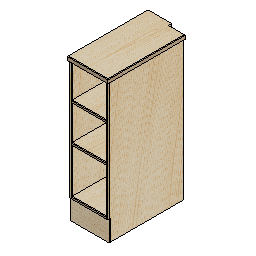
model (Autodesk Fusion 360 design; units mm, degrees)
Autodesk Fusion 360 part; units mm, degrees
note: some values were not read from the file. Chosen so that the rebuilt part matches the saved one: which bodies a step acts on.
sketch "cabinet" plane through (0, 0, 0) normal (1, 0, 0) x (0, 1, 0) in component "bounds"
  line L0 (0, 0) -> (0, 109)
  line L1 (0, 109) -> (-72, 109)
  line L2 (-72, 109) -> (-72, 884)
  line L3 (-72, 884) -> (413, 884)
  line L4 (413, 884) -> (413, 0)
  line L5 (413, 0) -> (0, 0)
  line L6 (-72, 884) -> (-102, 884)
  line L7 (-102, 884) -> (-102, 914)
  line L8 (-102, 914) -> (413, 914)
  line L9 (413, 914) -> (413, 884)
  dimension "d1" = 30
  dimension "d2" = 30
  dimension "d3" = 109
  dimension "d4" = 72
  dimension "d5" = 485
  dimension "d6" = 884
  constraint coincident L0.start L5.end
  constraint vertical L0
  constraint horizontal L1
  constraint vertical L2
  constraint horizontal L5
  constraint vertical L4
  constraint horizontal L3
  constraint vertical L9
  constraint horizontal L6
  constraint vertical L7
  constraint horizontal L8
  measures "d1" distance of L2.end L6.end
  measures "d2" distance of L6.end L7.end
  measures "d3" distance of L0.start L0.end
  measures "d4" distance of L0.end L1.end
  measures "d5" distance of L2 L4
  measures "d6" distance of L3.end L4.end
extrude "Extrude1" add sketch "cabinet" against normal blind 30 makes body 1 in component "bounds"
extrude "Extrude2" add sketch "cabinet" along normal blind 30 contours L3 L6 L7 L8 L9 bodies 1 in component "bounds"
sketch "wall" plane through (0, 413, 0) normal (0, 1, 0) x (-1, 0, 0) in component "bounds"
  line L0 (0, 884) -> (0, 0)
  line L1 (0, 0) -> (30, 0)
  line L2 (30, 0) -> (30, 914)
  line L3 (30, 914) -> (-30, 914)
  line L4 (-30, 914) -> (-30, 884)
  line L5 (-30, 884) -> (0, 884)
  line L6 (30, 914) -> (-205, 914)
  line L7 (-205, 914) -> (-205, 0)
  line L8 (-205, 0) -> (30, 0)
  line L9 (30, 0) -> (30, 914)
  line L10 (-127, 914) -> (-127, 95)
  line L11 (-127, 95) -> (0, 95)
  dimension "d11" = 78
  dimension "d13" = 95
  dimension "d14" = 205
  constraint horizontal L6
  constraint vertical L7
  constraint horizontal L8
  constraint vertical L9
  constraint coincident L2.end L3.start
  constraint coincident L0.end L8
  constraint coincident L6 L10.start
  constraint coincident L0 L11.end
  constraint vertical L10
  constraint horizontal L11
  measures "d11" distance of L7 L10
  measures "d13" distance of L8 L11
  measures "d14" distance of L0 L7
extrude "Extrude3" add sketch "wall" along normal blind 30 separate body makes body 2 in component "bounds"
extrude "Extrude4" add sketch "wall" against normal blind 18 contours L0 L6 L7 L8 L10 L11 bodies 2 in component "bounds"
sketch "bathtub" plane through (205, 0, 0) normal (1, 0, 0) x (0, 1, 0) in component "bounds"
  line L0 (395, 0) -> (443, 0)
  line L1 (443, 0) -> (443, 914)
  line L2 (443, 914) -> (395, 914)
  line L3 (395, 914) -> (395, 0)
  line L4 (443, 0) -> (-357, 0)
  line L5 (-357, 0) -> (-357, 520)
  line L6 (-357, 520) -> (443, 520)
  line L7 (443, 520) -> (443, 0)
  dimension "d19" = 520
  dimension "d20" = 800
  constraint horizontal L4
  constraint vertical L5
  constraint horizontal L6
  constraint vertical L7
  constraint coincident L0.end L1.start
  measures "d19" distance of L4.end L5.end
  measures "d20" distance of L0.end L4.end
extrude "Extrude5" add sketch "bathtub" along normal blind 30 separate body contours L0 L1 L3 L4 L6 L7 | L3 L4 L5 L6 makes body 3 in component "bounds"
extrude "Extrude6" add sketch "bathtub" along normal blind 30 contours L1 L2 L3 L6 bodies 2 in component "bounds"
sketch "face" plane through (0, 0, 0) normal (0, 1, 0) x (1, 0, 0) in component "unit"
  line L0 (0, 0) -> (205, 0)
  line L1 (205, 0) -> (205, -750)
  line L2 (205, -750) -> (0, -750)
  line L3 (0, -750) -> (0, 0)
  line L4 (9, -750) -> (9, 0)
  line L5 (196, -750) -> (196, 0)
  line L6 (9, -375) -> (0, -375) construction
  line L7 (205, -375) -> (196, -375) construction
  line L8 (0, -750) -> (0, -768)
  line L9 (0, -768) -> (217, -768)
  line L10 (205, -750) -> (217, -750)
  line L11 (217, -750) -> (217, -768)
  line L12 (9, -118) -> (196, -118)
  line L13 (196, -109) -> (9, -109)
  line L14 (0, -109) -> (-30, -109)
  line L15 (196, -109) -> (205, -109)
  line L16 (9, -109) -> (0, -109)
  line L17 (9, -563) -> (196, -563)
  line L18 (196, -554) -> (9, -554)
  line L19 (9, -367) -> (196, -367)
  line L20 (196, -358) -> (9, -358)
  dimension "d25" = 205
  dimension "d26" = 9
  dimension "d27" = 750
  dimension "d32" = 18
  dimension "d33" = 12
  dimension "d34" = 9
  dimension "d35" = 9
  dimension "d36" = 187
  dimension "d37" = 9
  dimension "d38" = 187
  dimension "d39" = 240
  constraint horizontal L0
  constraint vertical L1
  constraint horizontal L2
  constraint vertical L3
  constraint coincident L0.start L3.end
  constraint coincident L2 L4.start
  constraint coincident L2 L5.start
  constraint coincident L0 L5.end
  constraint vertical L4
  constraint vertical L5
  constraint coincident L0 L4.end
  constraint midpoint L4 L6.start
  constraint midpoint L3 L6.end
  constraint midpoint L1 L7.start
  constraint midpoint L5 L7.end
  constraint equal L6 L7
  constraint vertical L8
  constraint horizontal L9
  constraint horizontal L10
  constraint vertical L11
  constraint coincident L4 L12.start
  constraint coincident L5 L12.end
  constraint coincident L5 L13.start
  constraint coincident L4 L13.end
  constraint horizontal L13
  constraint horizontal L12
  constraint coincident L1 L15.end
  constraint perpendicular L1 L15
  constraint coincident L3 L14.start
  constraint perpendicular L3 L16
  constraint coincident L4 L17.start
  constraint coincident L5 L17.end
  constraint coincident L5 L18.start
  constraint coincident L4 L18.end
  constraint horizontal L18
  constraint horizontal L17
  constraint coincident L4 L19.start
  constraint coincident L5 L19.end
  constraint coincident L5 L20.start
  constraint coincident L4 L20.end
  constraint horizontal L20
  constraint horizontal L19
  constraint collinear L13 L14
  measures "d25" distance of L0.start L0.end
  measures "d26" distance of L6.start L6.end
  measures "d27" distance of L0.end L1.end
  measures "d32" distance of L2 L9
  measures "d33" distance of L1.end L10.end
  measures "d34" distance of L12 L13
  measures "d35" distance of L17 L18
  measures "d36" distance of L2 L17
  measures "d37" distance of L19 L20
  measures "d38" distance of L18 L19
  measures "d39" distance of L12 L20
extrude "Extrude1'" add sketch "face" along normal up to surface (413 mm away) and the other way blind 18 separate body contours L2 L8 L9 L10 L11 makes body 4 in component "unit"
combine "Combine1" operation cut target body 4 tool bodies 2 keep tools in component "unit"
extrude "Extrude2'" add sketch "face" against normal blind 9 from surface at 395 separate body contours L0 L4 L5 L13 | L4 L5 L12 L13 | L4 L5 L12 L20 | L2 L4 L5 L17 | L4 L5 L19 L20 | L4 L5 L17 L18 | L4 L5 L18 L19 makes body 5 in component "unit"
extrude "Extrude3'" add sketch "face" along normal blind 9 separate body contours L0 L3 L4 L16 | L0 L4 L5 L13 | L0 L1 L5 L15 makes body 6 in component "unit"
extrude "Extrude4'" add sketch "face" along normal up to surface (395 mm away) separate body contours L0 L3 L4 L16 | L2 L3 L4 L16 | L0 L1 L5 L15 | L1 L2 L5 L15 makes body 7 at (205, 131.6667, 250) makes body 8 at (9, 131.6667, 500) in component "unit"
combine "Combine2" operation cut target body 7 tool bodies 6 keep tools in component "unit"
combine "Combine3" operation cut target body 8 tool bodies 6 keep tools in component "unit"
extrude "Extrude5'" add sketch "face" along normal up to surface (386 mm away) separate body contours L4 L5 L12 L13 | L4 L5 L19 L20 | L4 L5 L17 L18 makes body 9 at (133.6667, 257.3333, 554) makes body 10 at (133.6667, 257.3333, 358) makes body 11 at (133.6667, 257.3333, 109) in component "unit"
extrude "Extrude6'" add sketch "face" against normal blind 6 separate body contours L2 L3 L4 L16 | L1 L2 L5 L15 makes body 12 at (199, 0, 322.6667) makes body 13 at (3, 0, 536.3333) in component "unit"
extrude "Extrude7" add 3 faces at (71.3333, 0, 557) (71.3333, 0, 361) (71.3333, 0, 112) along direction (0, -1, 0) blind 6 separate body on bodies 9 10 11 makes body 14 at (71.3333, 0, 361) makes body 15 at (71.3333, 0, 557) makes body 16 at (71.3333, 0, 112) in component "unit"
sketch "top edge" plane through (0, 0, 768) normal (0, 0, 1) x (-1, 0, 0) in component "unit"
  line L0 (-217, -395) -> (-127, -395)
  line L1 (-127, -395) -> (-127, -413)
  line L2 (-127, -413) -> (0, -413)
  line L3 (0, -413) -> (0, 18)
  line L4 (0, 18) -> (-217, 18)
  line L5 (-217, 18) -> (-217, -395)
  line L6 (0, 12) -> (-211, 12)
  line L7 (-211, 12) -> (-211, -395)
  dimension "d56" = 6
  dimension "d57" = 6
  constraint coincident L3 L6.start
  constraint coincident L0 L7.end
  constraint horizontal L6
  constraint vertical L7
  measures "d56" distance of L5 L7
  measures "d57" distance of L4 L6
split "Split1" by curves path "top edge" along L6 L7 bodies 4 makes body 17 at (217, 119.6667, 756) in component "unit"
sketch "Sketch1" plane through (0, 0, 0) normal (0, 0, 1) x (1, 0, 0) in component "cutlist"
  line L0 (505, 0) -> (2031, 0)
  line L1 (2031, 0) -> (2031, 505)
  line L2 (2031, 505) -> (505, 505)
  line L3 (505, 505) -> (505, 0)
  line L4 (2031, 525) -> (2031, 1030)
  line L5 (2031, 1030) -> (505, 1030)
  line L6 (505, 1030) -> (505, 525)
  line L7 (505, 525) -> (2031, 525)
  line L8 (2031, 1050) -> (2031, 1555)
  line L9 (2031, 1555) -> (505, 1555)
  line L10 (505, 1555) -> (505, 1050)
  line L11 (505, 1050) -> (2031, 1050)
  line L12 (0, 0) -> (505, 0) construction
  line L13 (514.772, 400.776) -> (1264.772, 400.776) construction
  line L14 (1264.772, 400.776) -> (1264.772, 5.776) construction
  line L15 (1264.772, 5.776) -> (514.772, 5.776) construction
  line L16 (514.772, 5.776) -> (514.772, 400.776) construction
  line L17 (2024.772, 5.776) -> (1274.772, 5.776) construction
  line L18 (1274.772, 5.776) -> (1274.772, 400.776) construction
  line L19 (2024.772, 400.776) -> (2024.772, 5.776) construction
  line L20 (1274.772, 400.776) -> (2024.772, 400.776) construction
  line L21 (507.0464, 912.7813) -> (694.0464, 912.7813) construction
  line L22 (694.0464, 912.7813) -> (694.0464, 526.7813) construction
  line L23 (694.0464, 526.7813) -> (507.0464, 526.7813) construction
  line L24 (507.0464, 526.7813) -> (507.0464, 912.7813) construction
  line L25 (1382.278, 722.1268) -> (2023.278, 722.1268) construction
  line L26 (2023.278, 722.1268) -> (2023.278, 535.1268) construction
  line L27 (2023.278, 535.1268) -> (1382.278, 535.1268) construction
  line L28 (1382.278, 535.1268) -> (1382.278, 722.1268) construction
  line L29 (512.3437, 1029.9816) -> (717.3437, 1029.9816) construction
  line L30 (717.3437, 1029.9816) -> (717.3437, 920.9816) construction
  line L31 (717.3437, 920.9816) -> (512.3437, 920.9816) construction
  line L32 (512.3437, 920.9816) -> (512.3437, 1029.9816) construction
  line L33 (699.5464, 526.7813) -> (699.5464, 912.7813) construction
  line L34 (699.5464, 912.7813) -> (886.5464, 912.7813) construction
  line L35 (886.5464, 912.7813) -> (886.5464, 526.7813) construction
  line L36 (886.5464, 526.7813) -> (699.5464, 526.7813) construction
  line L37 (892.0464, 526.7813) -> (892.0464, 912.7813) construction
  line L38 (892.0464, 912.7813) -> (1079.0464, 912.7813) construction
  line L39 (1079.0464, 912.7813) -> (1079.0464, 526.7813) construction
  line L40 (1079.0464, 526.7813) -> (892.0464, 526.7813) construction
  dimension "d60" = 1526
  dimension "d64" = 0
  dimension "d65" = 1050
  dimension "d66" = 505
  dimension "d67" = 750
  dimension "d68" = 395
  dimension "d71" = 760
  dimension "d72" = 0
  dimension "d73" = 187
  dimension "d74" = 386
  dimension "d75" = 641
  dimension "d85" = 109
  dimension "d89" = 385
  dimension "d90" = 0
  dimension "d91" = 205
  constraint horizontal L0
  constraint vertical L1
  constraint horizontal L2
  constraint vertical L3
  constraint coincident L12.start origin
  constraint horizontal L12
  constraint equal L3 L12
  constraint horizontal L13
  constraint vertical L14
  constraint horizontal L15
  constraint vertical L16
  constraint horizontal L21
  constraint vertical L22
  constraint horizontal L23
  constraint vertical L24
  constraint horizontal L25
  constraint vertical L26
  constraint horizontal L27
  constraint vertical L28
  constraint horizontal L29
  constraint vertical L30
  constraint horizontal L31
  constraint vertical L32
  constraint equal L23 L28
  measures "d60" distance of L0.start L0.end
  measures "d66" distance of L0.end L1.end
  measures "d67" distance of L14.end L15.end
  measures "d68" distance of L13.start L15.end
  measures "d73" distance of L22.end L23.end
  measures "d74" distance of L21.start L23.end
  measures "d75" distance of L25.start L25.end
  measures "d85" distance of L29.start L31.end
  measures "d91" distance of L30 L32
component "bounds" placed x (1, 0, 0) y (0, 1, 0) z (0, 0, 1) at (0, 0, 0)
component "unit" placed x (1, 0, 0) y (0, 1, 0) z (0, 0, 1) at (0, 0, 0)
component "cutlist" placed x (1, 0, 0) y (0, 1, 0) z (0, 0, 1) at (0, 0, 0)
equation "d26 = caseT"
equation "caseT = 9 mm"
equation "topT = 18 mm"
equation "d32 = topT"
equation "d33 = d32 - edgeT"
equation "d34 = caseT"
equation "d35 = caseT"
equation "d37 = caseT"
equation "d42 = topT"
equation "d45 = -caseT"
equation "d47 = caseT"
equation "edgeT = 6 mm"
equation "d54 = -edgeT"
equation "d56 = edgeT"
equation "d57 = edgeT"
equation "d58 = edgeT"
named bodies: "cabinet", "wall", "bathtub"
